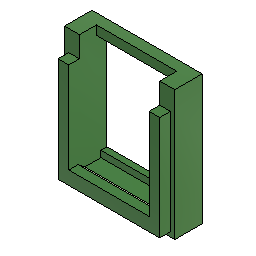
RJ45_EndCap_NEMA17 (Autodesk Fusion 360 archive; units mm, degrees)
design "RJ45_Panel_Adaptor"
Autodesk Fusion 360 part; units mm, degrees
sketch "Sketch1" plane through (0, 0, 0) normal (1, 0, 0) x (0, 1, 0)
  line L0 (7.123, -11.7) -> (7.123, 11.7)
  line L1 (0, 11.7) -> (0, -11.7)
  line L2 (7.123, -9) -> (6, -9)
  line L3 (6, -9) -> (6, -10.2)
  line L4 (6, -10.2) -> (3, -10.2)
  line L5 (7.123, 10) -> (5.173, 10)
  line L6 (5.173, 10) -> (5.173, 11.7)
  line L7 (7.123, 11.7) -> (0, 11.7)
  line L8 (3, -10.2) -> (1.747, -9.2)
  line L9 (0, -11.7) -> (7.123, -11.7)
  line L10 (0, -9.2) -> (1.747, -9.2)
  line L11 (0, 7.8) -> (2, 7.8)
  line L12 (2, 7.8) -> (2, 11.7)
  dimension "d2" = 7.123
  dimension "d3" = 1.7
  dimension "d4" = 1.95
  dimension "d5" = 1.123
  dimension "d6" = 3
  dimension "d11" = 1.2
  dimension "d36" = 1
  dimension "d37" = 141.407
  dimension "d38" = 1.5
  dimension "d39" = 9
  dimension "d92" = 2
  dimension "d93" = 19.5
  constraint coincident L0 L2.start
  constraint coincident L0 L5.start
  constraint coincident L6.end L7
  constraint vertical L1
  constraint horizontal L7
  constraint vertical L6
  constraint horizontal L5
  constraint vertical L0
  constraint horizontal L2
  constraint vertical L3
  constraint horizontal L4
  constraint perpendicular L0 L9
  constraint midpoint origin L1
  constraint coincident L1 L10.start
  constraint perpendicular L1 L10
  constraint coincident L1 L11.start
  constraint perpendicular L1 L11
  constraint coincident L7 L12.end
  constraint perpendicular L7 L12
  measures "d2" distance of L0.end L1.start
  measures "d3" distance of L5.end L6.end
  measures "d4" distance of L5.start L5.end
  measures "d5" distance of L2.start L2.end
  measures "d6" distance of L3.end L4.end
  measures "d11" distance of L2.end L3.end
  measures "d36" distance of L4 L10
  measures "d37" angle of L4 L8
  measures "d38" distance of L4 L9
  measures "d39" distance of origin L2
  measures "d92" distance of L11.start L11.end
  measures "d93" distance of L9 L11
extrude "Extrude1" add sketch "Sketch1" along normal mid plane 19 contours L0 L1 L2 L3 L4 L8 L9 L10 | L0 L5 L6 L7 makes body 1 at (-3.1667, 2.3743, -11.7) makes body 2 at (3.1667, 6.473, 11.7)
extrude "Extrude2" add sketch "Sketch1" along normal blind 2 from surface at -9.5 contours L0 L1 L2 L3 L4 L5 L6 L7 L8 L10 L11 L12 bodies 1 2
extrude "Extrude3" add sketch "Sketch1" against normal blind 2 from surface at 9.5 contours L0 L1 L2 L3 L4 L5 L6 L7 L8 L10 L11 L12 bodies 1
sketch "Sketch3" plane through (0, 0, 0) normal (0, 1, 0) x (1, 0, 0)
  line L0 (9.5, -7.8) -> (9.5, -11.7)
  line L1 (9.5, -11.7) -> (7.5, -11.7)
  line L2 (7.5, -7.8) -> (7.5, -10)
  line L3 (7.5, 9) -> (7.5, -7.8)
  line L4 (-7.5, 9) -> (7.5, 9)
  line L5 (-7.5, -10) -> (7.5, -10)
  line L6 (-7.5, -11.7) -> (7.5, -11.7)
  line L7 (-9.5, -11.7) -> (-9.5, -7.8)
  line L8 (-7.5, -10) -> (-7.5, -7.8)
  line L9 (-9.5, -11.7) -> (-7.5, -11.7)
  line L10 (-7.5, -7.8) -> (-7.5, 9)
  line L11 (-9.5, 11.7) -> (-9.5, -7.8)
  line L12 (9.5, 11.7) -> (-9.5, 11.7)
  line L13 (9.5, 11.7) -> (9.5, -7.8)
  line L14 (10.3, -7.936) -> (10.3, -12.564)
  line L15 (10.3, -12.564) -> (7.3, -12.564)
  line L16 (-7.3, -12.564) -> (7.3, -12.564)
  line L17 (-10.3, -12.564) -> (-7.3, -12.564)
  line L18 (-10.3, -12.564) -> (-10.3, -7.936)
  line L19 (-10.3, 12.564) -> (-10.3, -7.936)
  line L20 (-10.3, 12.564) -> (10.3, 12.564)
  line L21 (10.3, 12.564) -> (10.3, -7.936)
  line L22 (9.5, -11.7) -> (10.3, -11.7)
  line L23 (-9.5, -11.7) -> (-10.3, -11.7)
  circle A0 centre (0, 0) radius 1.9085
  constraint coincident L7.start L9.start
  constraint coincident L0.end L1.start
  constraint coincident L14 L22.end
  constraint perpendicular L14 L22
  constraint coincident L18 L23.end
  constraint perpendicular L18 L23
  constraint coincident A0.centre origin
extrude "Extrude5" add sketch "Sketch3" along normal up to surface (5.123 mm away) from surface at 2 contours L0 L7 L11 L12 L13 L14 L18 L19 L20 L21 L22 L23 bodies 1
